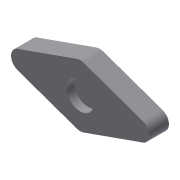
# Autodesk Inventor part: Part1
Saved by Autodesk Inventor 2015 (Build 190159000, 159)
## iProperties
Created: 2014-11-08
Part Number: Part1
Material: Generic
Document SubType Name: Modeling
Designer: Peter
Density: 1 g/cm^3
Appearance: Default
Author: Peter
Autodesk Inventor part; units mm, degrees
ref_plane "YZ Plane" through (0, 0, 0) normal (1, 0, 0) x (0, 1, 0)
ref_plane "XZ Plane" through (0, 0, 0) normal (0, 1, 0) x (-1, 0, 0)
ref_plane "XY Plane" through (0, 0, 0) normal (0, 0, 1) x (1, 0, 0)
sketch "Sketch1" plane through (0, 0, 0) normal (0, 0, 1) x (1, 0, 0)
  line L0 (1.0583, 9.7858) -> (20.2702, 2.9934)
  line L1 (20.2702, -2.9934) -> (1.0583, -9.7858)
  line L2 (-1.0583, -9.7858) -> (-20.2702, -2.9934)
  line L3 (-20.2702, 2.9934) -> (-1.0583, 9.7858)
  arc A0 (20.2702, -2.9934) -> (20.2702, 2.9934) centre (19.2118, 0) ccw
  arc A1 (-20.2702, 2.9934) -> (-20.2702, -2.9934) centre (-19.2118, 0) ccw
  arc A2 (1.0583, 9.7858) -> (-1.0583, 9.7858) centre (0, 6.7924) ccw
  arc A3 (-1.0583, -9.7858) -> (1.0583, -9.7858) centre (0, -6.7924) ccw
  point P0 (0, 10.16)
  point P1 (28.7368, 0)
  point P2 (0, -10.16)
  point P3 (-28.7368, 0)
  point P4 (0, 0)
  dimension "d0" = 30.48
  dimension "d1" = 20.32
  dimension "d2" = 3.175
  constraints: 8 end point, 8 point on circle, 8 point on line, 8 tangent, 4 centre point, 3 equal length, 3 equal radius, 2 horizontal alignment, 2 vertical alignment
  measures "d0" distance of point (0, 10.16) point (28.737, 0)
  measures "d1" distance of point (0, 10.16) point (0, -10.16)
  measures "d2" radius of A0
extrude "Extrusion1" add sketch "Sketch1" along normal blind 6.35
sketch "Sketch2" plane through (0, 0, 6.35) normal (0, 0, 1) x (1, 0, 0)
  circle A0 centre (0, 0) radius 4.4138
  constraints: 1 centre point
extrude "Extrusion2" cut sketch "Sketch2" against normal blind 2.54
body "Solid1"
